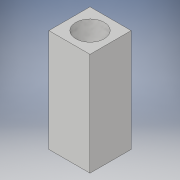
# Autodesk Inventor part: thumb
Saved by Autodesk Inventor 2018 (Build 220112000, 112)
## iProperties
Created: 2020-03-06
Part Number: thumb
Material: Generic
Document SubType Name: Modeling
Designer: Jesse R-B
Density: 1 g/cm^3
Appearance: Default
Author: Jesse R-B
Autodesk Inventor part; units mm, degrees
ref_plane "YZ Plane" through (0, 0, 0) normal (1, 0, 0) x (0, 1, 0)
sketch "Sketch1" plane through (0, 0, 0) normal (1, 0, 0) x (0, 1, 0)
  line L0 (0, 0) -> (76.2, 0)
  line L1 (76.2, 0) -> (76.2, -30.48)
  line L2 (76.2, -30.48) -> (0, -30.48)
  line L3 (0, -30.48) -> (0, 0)
  dimension "d0" = 30.48
  dimension "d1" = 76.2
  constraints: 8 end point, 2 parallel, 1 horizontal, 1 perpendicular
  measures "d0" distance of L0.end L1.end
  measures "d1" distance of L1.end L2.end
extrude "Extrusion1" add sketch "Sketch1" along normal blind 30.48
sketch "Sketch2" plane through (0, 76.2, 0) normal (0, 1, 0) x (1, 0, 0)
  line L0 (0, 0) -> (0, 30.48) projected
  line L1 (0, 0) -> (30.48, 0) projected
  line L2 (30.48, 30.48) -> (30.48, 0) projected
  line L3 (0, 30.48) -> (30.48, 30.48) projected
  circle A0 centre (15.24, 15.24) radius 10.541
  point P0 (0, 0)
  dimension "d4" = 21.082
  dimension "d5" = 15.24
  dimension "d6" = 15.24
  constraints: 1 centre point
  measures "d4" diameter of A0
  measures "d5" distance from line of L0 A0.centre
  measures "d6" distance from line of L1 A0.centre
extrude "Extrusion2" cut sketch "Sketch2" against normal through all contours A0
ref_plane "Work Plane1" through (15.24, 0, 0) normal (1, 0, 0) x (0, 0, -1)
ref_plane "Work Plane2" through (0, 38.1, 0) normal (0, 1, 0) x (1, 0, 0)
body "Solid1"
